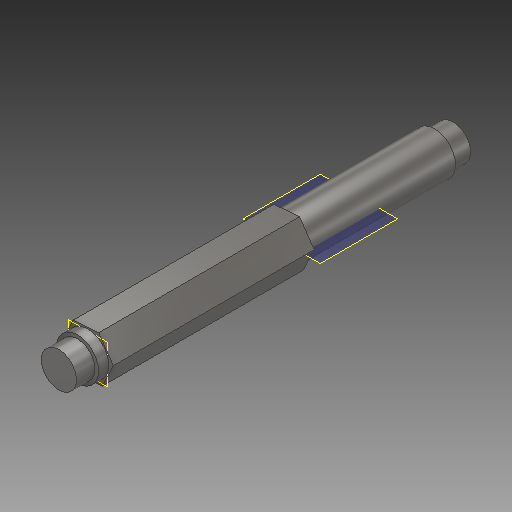
# Autodesk Inventor part: Mecanum Axle
Saved by Autodesk Inventor 2019 (Build 230136000, 136)
## iProperties
Created: 2019-11-02
Part Number: Mecanum Axle
Material: Stainless Steel
Document SubType Name: Modeling
Designer: admin
Density: 8 g/cm^3
Appearance: Semi-Polished
Mass: 109.71 g
Surface Area: 48.9651 cm^2
Volume: 13.7138 cm^3
Author: admin
Autodesk Inventor part; units mm, degrees
ref_plane "YZ Plane" through (0, 0, 0) normal (1, 0, 0) x (0, 1, 0)
ref_plane "XZ Plane" through (0, 0, 0) normal (0, 1, 0) x (-1, 0, 0)
ref_plane "XY Plane" through (0, 0, 0) normal (0, 0, 1) x (1, 0, 0)
sketch "Sketch1" plane through (0, 0, 0) normal (1, 0, 0) x (0, 1, 0)
  line L0 (5, 0) -> (5, -5.3)
  line L1 (5, -106.9) -> (5, -112.2)
  line L2 (5, -112.2) -> (0, -112.2)
  line L3 (0, -112.2) -> (0, 0)
  line L4 (0, 0) -> (5, 0)
  line L5 (5, -106.9) -> (6, -106.9)
  line L6 (6, -106.9) -> (6, -5.3)
  line L7 (6, -5.3) -> (5, -5.3)
  dimension "d2" = 5
  dimension "d3" = 5.3
  dimension "d4" = 5.3
  dimension "d6" = 112.2
  dimension "d16" = 6
  dimension "d17" = 5
  constraints: 16 end point, 5 perpendicular, 1 coincident, 1 horizontal, 1 vertical
  measures "d2" distance of L3.end L0.start
  measures "d3" distance of L0.start L0.end
  measures "d4" distance of L1.start L1.end
  measures "d6" distance of L2.end L3.end
  measures "d16" distance between parallel lines of L3 L6
  measures "d17" distance between parallel lines of L3 L1
revolve "Revolution1" add sketch "Sketch1" angle 360 about axis through (0, 0, -112.2) along (0, 0, 1)
ref_plane "Work Plane1" through (0, 0, -74.4) normal (0, -1, 0) x (1, 0, 0)
sketch "Sketch3" plane through (0, 0, -74.4) normal (0, -1, 0) x (1, 0, 0)
  circle A0 centre (0, -22.2) radius 2.65
  line L0 (-5, -37.8) -> (5, -37.8) projected
  line L1 (0, -22.2) -> (0, -37.8) construction
  point P0 (0, 74.4)
  dimension "d12" = 5.3
  dimension "d13" = 15.6
  constraints: 2 end point, 1 centre point, 1 midpoint, 1 vertical
  measures "d12" diameter of A0
  measures "d13" distance from line of L0 L1.start
extrude "Extrusion2" cut sketch "Sketch3" along normal blind 10
ref_plane "Work Plane4" through (0, 0, -8.2) normal (0, 0, 1) x (1, 0, 0)
sketch "Sketch5" plane through (-142.34, -16.1386, -8.2) normal (0, 0, 1) x (-0.9033, 0.429, 0)
  line L0 (-121.6494, -68.3151) -> (-115.2993, -71.9814)
  line L1 (-115.2993, -71.9814) -> (-115.2993, -79.3139)
  line L2 (-115.2993, -79.3139) -> (-121.6494, -82.9801)
  line L3 (-121.6494, -82.9801) -> (-127.9995, -79.3139)
  line L4 (-127.9995, -79.3139) -> (-127.9995, -71.9814)
  line L5 (-127.9995, -71.9814) -> (-121.6494, -68.3151)
  line L6 (-121.6494, -82.9801) -> (-121.6494, -68.3151) construction
  point P0 (-121.6494, -75.6476)
  point P1 (-121.6494, -75.6476)
  dimension "d21" = 14.665
  constraints: 14 end point, 1 coincident, 13 other
  measures "d21" distance of L2.end L0.start
extrude "Extrusion4" add sketch "Sketch5" against normal blind 57.15
body "Solid1"
